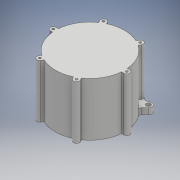
# Autodesk Inventor part: Motor
Saved by Autodesk Inventor 2018 (Build 220112000, 112)
## iProperties
Created: 2017-06-08
Part Number: Motor
Material: Generic
Document SubType Name: Modeling
Designer: eroldan
Density: 1 g/cm^3
Appearance: Default
Author: eroldan
Autodesk Inventor part; units mm, degrees
ref_plane "YZ Plane" through (0, 0, 0) normal (1, 0, 0) x (0, 1, 0)
ref_plane "XZ Plane" through (0, 0, 0) normal (0, 1, 0) x (-1, 0, 0)
ref_plane "XY Plane" through (0, 0, 0) normal (0, 0, 1) x (1, 0, 0)
sketch "Sketch1" plane through (0, 0, 0) normal (0, 0, 1) x (1, 0, 0)
  circle A0 centre (0, 0) radius 66 construction
  line L0 (-33, 57.1577) -> (33, 57.1577) construction
  circle A1 centre (-33, 57.1577) radius 19.5 construction
  circle A2 centre (33, 57.1577) radius 19.5 construction
  line L1 (-52, 52.7702) -> (52, 52.7702) construction
  line L2 (-33, 57.1577) -> (0, 0) construction
  line L3 (-28.4534, 59.7827) -> (-26.342, 56.1257)
  line L4 (-37.5466, 54.5327) -> (-35.4353, 50.8757)
  arc A3 (-28.3526, 59.5998) -> (-37.4386, 54.3539) centre (-33, 57.1577) ccw
  line L5 (0, 0) -> (52, 52.7702) construction
  arc A4 (56.6299, 48.2079) -> (48.2525, 58.0812) centre (52, 52.7702) ccw
  line L6 (56.6299, 48.2079) -> (50.3646, 41.8498)
  arc A5 (37.3563, 60.0877) -> (48.2525, 58.0812) centre (43.7855, 64.4119) ccw
  arc A6 (37.3563, 60.0877) -> (28.4534, 59.7827) centre (33, 57.1577) ccw
  line L7 (26.342, 56.1257) -> (28.4534, 59.7827)
  line L8 (17.0312, 21.5298) -> (26.342, 56.1257)
  arc A7 (45.4607, 42.1583) -> (49.9886, 36.6761) centre (0, 0) ccw construction
  arc A8 (50.3646, 41.8498) -> (49.9886, 36.6761) centre (53.2137, 39.0423) ccw
  line L9 (49.9886, 36.6761) -> (17.0312, 21.5298)
  arc A9 (-26.342, 56.1257) -> (-35.4353, 50.8757) centre (0, 0) ccw
  circle A10 centre (0, 0) radius 62
  dimension "d3" = 19.5
  dimension "d1" = 66
  dimension "d2" = 132
  dimension "d4" = 19.5
  dimension "d6" = 104
  dimension "d40" = 13
  dimension "d43" = 10.5
  dimension "d44" = 5.25
  dimension "d45" = 7.7481
  dimension "d46" = 4
  dimension "d67" = 4
  constraints: 24 point on circle, 20 end point, 10 centre point, 7 coincident, 7 tangent, 3 parallel, 2 concentric, 2 horizontal, 3 other
  measures "d1" distance of L0.start L0.end
  measures "d2" diameter of A0
  measures "d4" radius of A2
  measures "d6" distance of L1.start L1.end
  measures "d40" diameter of A4
  measures "d43" diameter of A3
  measures "d44" radius of A6
  measures "d45" radius of A5
  measures "d46" radial gap between concentric circles of A0 A7
  measures "d67" radius of A8
extrude "Extrusion5" add sketch "Sketch1" along normal mid plane 11 contours A10 L9 L8 | L7 A6 A5 A4 L6 A8 A10
extrude "Extrusion6" add sketch "Sketch1" along normal mid plane 11 contours L3 A9 L4 A3
hole "Hole3" at (-33, 57.1577, 0) at (-52, 52.7702, 0) at (33, 57.1577, 0) direction (0, 0, -1) diameter 4 end through all both
hole "Hole4" at (52, 52.7702, 0) direction (0, 0, -1) diameter 8 end through all both
pattern_circular "Circular Pattern1" count 6 over 360 about axis through (0, 0, -10) along (0, 0, 1) of "Extrusion6", "Hole3"
mirror "Mirror1" about plane through (0, 0, 0) normal (1, 0, 0) of "Extrusion5", "Hole4", "Extrusion6", "Hole3", "Circular Pattern1"
extrude "Extrusion7" add sketch "Sketch1" along normal mid plane 11 contours A10 L8 L9 A9 | A10 L9 L8
sketch "Sketch2" plane through (0, 0, 5.5) normal (0, 0, 1) x (1, 0, 0)
  line L0 (-61.7773, 40.0924) -> (61.7773, 40.0924)
  line L1 (61.7773, 40.0924) -> (61.7773, 80.3948)
  line L2 (61.7773, 80.3948) -> (-61.7773, 80.3948)
  line L3 (-61.7773, 80.3948) -> (-61.7773, 40.0924)
  line L4 (-61.7773, 40.0924) -> (61.7773, 80.3948) construction
  line L5 (61.7773, 40.0924) -> (-61.7773, 80.3948) construction
  circle A0 centre (-45.2667, 68.1507) radius 4.75 construction
  line L6 (0, 0) -> (0, 86.0303)
  circle A1 centre (-52, 52.7702) radius 4 projected
  circle A2 centre (52, 52.7702) radius 4 projected
  circle A3 centre (33, 57.1577) radius 2 projected
  circle A4 centre (-33, 57.1577) radius 2 projected
  point P0 (0, 60.2436)
  point P1 (0, 60.2436)
  point P2 (45.2667, 68.1507)
  point P3 (-61.7773, -5.25)
  dimension "d78" = 9.5
  constraints: 14 end point, 3 midpoint, 2 parallel, 2 vertical alignment, 1 centre point, 1 coincident, 1 horizontal, 1 perpendicular, 1 symmetric about line, 1 vertical
  measures "d78" diameter of A0
extrude "Extrusion8" add sketch "Sketch2" along normal blind 3.7 separate body contours L3 L2 L6 L0 | L6 L2 L1 L0 | A1 | A2 | A3 | A4
hole "Hole8" at (-45.2667, 68.1507, 5.5) at (45.2667, 68.1507, 5.5) direction (0, 0, 1) diameter 9.5 end through all both bodies 1 2
hole "Hole9" at (-52, 52.7702, 5.5) at (52, 52.7702, 5.5) direction (0, 0, -1) diameter 8.5 end through all both bodies 2
hole "Hole10" at (-33, 57.1577, 5.5) at (33, 57.1577, 5.5) direction (0, 0, -1) diameter 4.5 end through all both bodies 2
fillet "Fillet1" radius 15 2 edges at (-61.7773, 80.3948, 7.35) (61.7773, 80.3948, 7.35)
fillet "Fillet1" radius 10 2 edges at (-61.7773, 40.0924, 7.35) (61.7773, 40.0924, 7.35)
sketch "Sketch4" plane through (0, 0, -5.5) normal (0, 0, -1) x (-1, 0, 0)
  circle A0 centre (0, 0) radius 57 construction
  line L0 (51.7773, 40.0924) -> (-51.7773, 40.0924) construction
  arc A1 (40.5166, 40.0924) -> (-40.5166, 40.0924) centre (0, 0) ccw
  line L1 (-46.7773, 80.3948) -> (46.7773, 80.3948) projected
  arc A2 (-46.7773, 80.3948) -> (-61.7773, 65.3948) centre (-46.7773, 65.3948) ccw projected
  line L2 (-61.7773, 50.0924) -> (-61.7773, 65.3948) projected
  arc A3 (-61.7773, 50.0924) -> (-51.7773, 40.0924) centre (-51.7773, 50.0924) ccw projected
  arc A4 (51.7773, 40.0924) -> (61.7773, 50.0924) centre (51.7773, 50.0924) ccw projected
  line L3 (61.7773, 65.3948) -> (61.7773, 50.0924) projected
  arc A5 (61.7773, 65.3948) -> (46.7773, 80.3948) centre (46.7773, 65.3948) ccw projected
  line L4 (51.7773, 40.0924) -> (-51.7773, 40.0924) construction
  line L5 (-51.7773, 40.0924) -> (-40.5166, 40.0924)
  line L6 (51.7773, 40.0924) -> (40.5166, 40.0924)
  circle A6 centre (-45.2667, 68.1507) radius 4.75 projected
  circle A7 centre (-33, 57.1577) radius 2 projected
  circle A8 centre (45.2667, 68.1507) radius 4.75 projected
  circle A9 centre (33, 57.1577) radius 2 projected
  dimension "d126" = 114
  constraints: 4 end point, 4 point on circle, 2 centre point, 2 collinear, 1 coincident, 1 concentric
  measures "d126" diameter of A0
extrude "Extrusion10" add sketch "Sketch4" along normal blind 3.7 separate body
sketch "Sketch7" plane through (0, 0, 5.5) normal (0, 0, 1) x (1, 0, 0)
  circle A0 centre (0, 0) radius 62 projected
  arc A1 (66, -5.25) -> (66, 5.25) centre (66, 0) ccw projected
  line L0 (66, 5.25) -> (61.7773, 5.25) projected
  line L1 (61.7773, -5.25) -> (66, -5.25) projected
  line L2 (28.4534, 59.7827) -> (26.342, 56.1257) projected
  arc A2 (37.3563, 60.0877) -> (28.4534, 59.7827) centre (33, 57.1577) ccw projected
  line L3 (-26.342, 56.1257) -> (-28.4534, 59.7827) projected
  arc A3 (-28.4534, 59.7827) -> (-37.3563, 60.0877) centre (-33, 57.1577) ccw projected
  line L4 (-61.7773, 5.25) -> (-66, 5.25) projected
  arc A4 (-66, 5.25) -> (-66, -5.25) centre (-66, 0) ccw projected
  line L5 (-66, -5.25) -> (-61.7773, -5.25) projected
  line L6 (-28.4534, -59.7827) -> (-26.342, -56.1257) projected
  arc A5 (-37.5466, -54.5327) -> (-28.4534, -59.7827) centre (-33, -57.1577) ccw projected
  line L7 (-35.4353, -50.8757) -> (-37.5466, -54.5327) projected
  line L8 (26.342, -56.1257) -> (28.4534, -59.7827) projected
  arc A6 (28.4534, -59.7827) -> (37.5466, -54.5327) centre (33, -57.1577) ccw projected
  line L9 (37.5466, -54.5327) -> (35.4353, -50.8757) projected
  circle A7 centre (-33, 57.1577) radius 2 projected
  arc A8 (-28.4534, 59.7827) -> (-37.3563, 60.0877) centre (-33, 57.1577) ccw projected
  arc A9 (-28.4534, 59.7827) -> (-37.5466, 54.5327) centre (-33, 57.1577) ccw
  line L10 (-37.5466, 54.5327) -> (-35.4353, 50.8757)
  arc A10 (37.5466, 54.5327) -> (37.3563, 60.0877) centre (33, 57.1577) ccw
  line L11 (37.5466, 54.5327) -> (35.4353, 50.8757)
  circle A11 centre (-66, 0) radius 2 projected
  circle A12 centre (33, 57.1577) radius 2 projected
  circle A13 centre (66, 0) radius 2 projected
  circle A14 centre (33, -57.1577) radius 2 projected
  circle A15 centre (-33, -57.1577) radius 2 projected
  point P0 (0, 0)
  constraints: 4 end point, 4 point on circle, 2 centre point, 2 coincident, 2 parallel, 3 other
extrude "Extrusion12" add sketch "Sketch7" along normal blind 85 bodies 1
sketch "Sketch8" plane through (0, 0, -5.5) normal (0, 0, -1) x (-1, 0, 0)
  circle A0 centre (0, 0) radius 25
  dimension "d135" = 50
  constraints: 1 centre point, 1 coincident
  measures "d135" diameter of A0
extrude "Extrusion13" add sketch "Sketch8" along normal blind 5 bodies 1
sketch "Sketch9" plane through (0, 0, -10.5) normal (0, 0, -1) x (-1, 0, 0)
  circle A0 centre (0, 0) radius 6
  dimension "d138" = 12
  constraints: 1 centre point, 1 coincident
  measures "d138" diameter of A0
extrude "Extrusion14" add sketch "Sketch9" along normal blind 22.5 bodies 1
sketch "Sketch10" plane through (0, 0, -5.5) normal (0, 0, -1) x (-1, 0, 0)
  circle A0 centre (66, 0) radius 2 projected
  point P0 (0, 0)
  point P1 (45, 0)
  point P2 (0, 0)
  point P3 (0, -45)
  point P4 (-45, 0)
  dimension "d141" = 21
  dimension "d151" = 180
  constraints: 1 coincident, 3 other
  measures "d141" distance of point (45, 0) A0.centre
hole "Hole11" at (-45, 0, -5.5) at (0, -45, -5.5) at (45, 0, -5.5) direction (0, 0, 1) diameter 6 depth 12 tip angle 118 bodies 1
equation "\"d3\" = d4"
body "Solid2"
body "Solid3"
body "Solid4"
